Autodesk Inventor part; units mm, degrees
(part 5 of 6)
sketch "S12_252p5" plane through (0, 0, 0) normal (0, 0, 1) x (1, 0, 0)
  spline S0 degree 4 poles (166.9793, -57.9524) (166.9462, -57.9325) (166.7851, -57.8344) (166.5141, -57.6708) (166.0568, -57.3944) (165.5757, -57.1034) (164.9842, -56.7476) (164.2877, -56.3279) (163.4842, -55.8462) (162.5759, -55.3021) (161.5628, -54.6978) (160.4459, -54.033) (159.2262, -53.3098) (157.9042, -52.5289) (156.4819, -51.6916) (154.959, -50.7997) (153.338, -49.8542) (151.6196, -48.8571) (149.8054, -47.8089) (147.8966, -46.7125) (145.8951, -45.5691) (143.8025, -44.3805) (141.6201, -43.1481) (139.3507, -41.8743) (136.9951, -40.5607) (134.5563, -39.2099) (132.0355, -37.8225) (129.4358, -36.4019) (126.7586, -34.949) (124.007, -33.4672) (121.1827, -31.9571) (118.2887, -30.4221) (115.3274, -28.8634) (112.3016, -27.2839) (109.2136, -25.6852) (106.0671, -24.0697) (102.8636, -22.4398) (99.6073, -20.7974) (96.3005, -19.1452) (92.9462, -17.4849) (89.5478, -15.8193) (86.108, -14.1502) (82.6304, -12.4799) (79.1182, -10.811) (75.574, -9.1458) (72.0022, -7.4865) (68.4051, -5.8346) (64.7867, -4.1941) (61.15, -2.5653) (57.4989, -0.952) (53.8362, 0.6448) (50.1662, 2.222) (46.4912, 3.7772) (42.8159, 5.3099) (39.1427, 6.8159) (35.4729, 8.2959) (31.8154, 9.7442) (28.1539, 11.1682) (24.4959, 12.5514) (20.856, 13.8924) (17.2349, 15.189) (13.6386, 16.4388) (10.0712, 17.6417) (6.5362, 18.794) (3.0374, 19.8976) (-0.4212, 20.9484) (-3.8363, 21.9476) (-7.2038, 22.8929) (-10.5204, 23.7851) (-13.7822, 24.6219) (-16.9859, 25.4043) (-20.1277, 26.131) (-23.204, 26.8025) (-26.2119, 27.4178) (-29.1474, 27.978) (-32.0075, 28.4823) (-34.7892, 28.9318) (-37.4891, 29.3257) (-40.1042, 29.666) (-42.6316, 29.9518) (-45.0687, 30.184) (-47.4123, 30.3643) (-49.6602, 30.492) (-51.8096, 30.5686) (-53.8586, 30.5956) (-55.8044, 30.5726) (-57.6453, 30.5014) (-59.3792, 30.3829) (-61.0045, 30.2176) (-62.5192, 30.0064) (-63.9224, 29.7508) (-65.2124, 29.4515) (-66.3881, 29.1083) (-67.4495, 28.7237) (-68.3947, 28.2959) (-69.2243, 27.8264) (-69.9371, 27.3151) (-70.5323, 26.7606) (-71.007, 26.1624) (-71.3603, 25.5232) (-71.5883, 24.8429) (-71.6921, 24.1329) (-71.6666, 23.4034) (-71.5144, 22.6557) (-71.2376, 21.8925) (-70.8384, 21.1138) (-70.3185, 20.32) (-69.6791, 19.5098) (-68.9214, 18.6836) (-68.046, 17.8415) (-67.0539, 16.9836) (-65.9464, 16.1108) (-64.7243, 15.223) (-63.3893, 14.3214) (-61.9425, 13.406) (-60.3859, 12.4783) (-58.7208, 11.5376) (-56.9491, 10.5863) (-55.0727, 9.6235) (-53.0939, 8.6504) (-51.014, 7.6678) (-48.8358, 6.6768) (-46.5615, 5.676) (-44.1931, 4.6688) (-41.7338, 3.6529) (-39.1849, 2.6307) (-36.5503, 1.6015) (-33.832, 0.5658) (-31.0327, -0.4749) (-28.1557, -1.5226) (-25.2032, -2.5742) (-22.1791, -3.6324) (-19.0858, -4.6945) (-15.9263, -5.762) (-12.7047, -6.8345) (-9.4228, -7.9111) (-6.0855, -8.9929) (-2.695, -10.0789) (0.7449, -11.1692) (4.2307, -12.2643) (7.7587, -13.3643) (11.3259, -14.4678) (14.9302, -15.5774) (18.5666, -16.6895) (22.2391, -17.8119) (25.9566, -18.935) (29.6926, -20.0539) (33.4519, -21.1684) (37.2253, -22.2781) (41.0102, -23.3826) (44.8023, -24.4815) (48.5975, -25.5737) (52.392, -26.6597) (56.1823, -27.7377) (59.9639, -28.809) (63.7335, -29.871) (67.4868, -30.9251) (71.22, -31.9694) (74.9301, -33.0031) (78.6119, -34.0269) (82.2628, -35.0388) (85.8789, -36.0381) (89.4562, -37.0254) (92.9912, -37.9982) (96.4806, -38.9572) (99.9205, -39.9007) (103.3076, -40.8281) (106.6385, -41.7385) (109.9101, -42.6317) (113.1182, -43.5064) (116.2605, -44.3616) (119.3336, -45.1966) (122.3339, -46.0115) (125.2589, -46.8038) (128.1054, -47.5746) (130.8706, -48.3216) (133.5514, -49.0456) (136.1456, -49.7442) (138.65, -50.4184) (141.0622, -51.0663) (143.3799, -51.6882) (145.6004, -52.2825) (147.7216, -52.8503) (149.7413, -53.389) (151.6572, -53.9) (153.4675, -54.382) (155.1703, -54.8341) (156.7635, -55.2571) (158.2458, -55.6502) (159.6155, -56.0123) (160.8707, -56.3443) (162.0109, -56.6449) (163.0338, -56.915) (163.9393, -57.1532) (164.7255, -57.3602) (165.3927, -57.5359) (165.9368, -57.6783) (166.4534, -57.8147) (166.7596, -57.8945) (166.942, -57.9424) (166.9793, -57.9524) knots 0 0 0 0 0 0.003306 0.005253 0.00752 0.010062 0.01285 0.015861 0.019079 0.022488 0.026078 0.029837 0.033757 0.037828 0.042045 0.046398 0.050884 0.055494 0.060224 0.065069 0.070023 0.075082 0.080241 0.085495 0.090841 0.096274 0.101791 0.107386 0.113057 0.118799 0.124609 0.130484 0.136419 0.142412 0.148458 0.154554 0.160697 0.166884 0.17311 0.179374 0.185671 0.191998 0.198352 0.20473 0.211128 0.217543 0.223972 0.230412 0.23686 0.243312 0.249765 0.256217 0.262663 0.2691 0.275526 0.281941 0.288345 0.294734 0.301105 0.307451 0.313767 0.320049 0.326294 0.332498 0.338659 0.344773 0.350837 0.356848 0.362801 0.368695 0.374525 0.380288 0.38598 0.391599 0.39714 0.4026 0.407976 0.413263 0.418458 0.423557 0.428556 0.433452 0.438241 0.442917 0.447478 0.451919 0.456236 0.460425 0.464482 0.468403 0.472185 0.475825 0.479322 0.482675 0.485889 0.48897 0.49193 0.494788 0.497572 0.50031 0.503032 0.505769 0.508552 0.511409 0.514365 0.517441 0.520647 0.523991 0.527474 0.531098 0.534861 0.538758 0.542789 0.546947 0.551231 0.555634 0.560154 0.564786 0.569527 0.574371 0.579315 0.584356 0.58949 0.594712 0.60002 0.605409 0.610877 0.61642 0.622034 0.627716 0.633463 0.639271 0.645138 0.651061 0.657035 0.663059 0.669128 0.675241 0.681393 0.687582 0.693804 0.700057 0.706341 0.712655 0.718998 0.725365 0.731751 0.738149 0.744556 0.750969 0.757385 0.7638 0.770211 0.776616 0.783011 0.789393 0.795759 0.802106 0.808429 0.814727 0.820996 0.827232 0.833433 0.839595 0.845714 0.851788 0.857813 0.863785 0.869702 0.875558 0.881352 0.887078 0.892735 0.898316 0.90382 0.909242 0.914577 0.919822 0.924972 0.930023 0.93497 0.939808 0.944533 0.949139 0.95362 0.95797 0.962183 0.966252 0.970169 0.973927 0.977515 0.980924 0.984141 0.987151 0.989939 0.99248 0.994747 0.996694 1 1 1 1 1
  circle A0 centre (0, 0) radius 5.15
  line L0 (-56.62, 15.9) -> (-46.42, 15.9)
  line L1 (-46.42, 15.9) -> (-46.42, 20.1)
  line L2 (-46.42, 20.1) -> (-56.62, 20.1)
  line L3 (-56.62, 20.1) -> (-56.62, 15.9)
  line L4 (-56.62, 15.9) -> (-46.42, 20.1) construction
  line L5 (-46.42, 15.9) -> (-56.62, 20.1) construction
  line L6 (-30.35, 13.1) -> (-20.15, 13.1)
  line L7 (-20.15, 13.1) -> (-20.15, 8.9)
  line L8 (-20.15, 8.9) -> (-30.35, 8.9)
  line L9 (-30.35, 8.9) -> (-30.35, 13.1)
  line L10 (-30.35, 13.1) -> (-20.15, 8.9) construction
  line L11 (-20.15, 13.1) -> (-30.35, 8.9) construction
  line L12 (64.9, -14.9) -> (75.1, -14.9)
  line L13 (75.1, -14.9) -> (75.1, -19.1)
  line L14 (75.1, -19.1) -> (64.9, -19.1)
  line L15 (64.9, -19.1) -> (64.9, -14.9)
  line L16 (64.9, -14.9) -> (75.1, -19.1) construction
  line L17 (75.1, -14.9) -> (64.9, -19.1) construction
  line L18 (29.9, -6.2) -> (40.1, -6.2)
  line L19 (40.1, -6.2) -> (40.1, -10.4)
  line L20 (40.1, -10.4) -> (29.9, -10.4)
  line L21 (29.9, -10.4) -> (29.9, -6.2)
  line L22 (29.9, -6.2) -> (40.1, -10.4) construction
  line L23 (40.1, -6.2) -> (29.9, -10.4) construction
  point P0 (166.7636, -57.8216)
  point P1 (166.4938, -57.6585)
  point P2 (166.1167, -57.4306)
  point P3 (165.6324, -57.138)
  point P4 (165.041, -56.7817)
  point P5 (164.3433, -56.3618)
  point P6 (163.5394, -55.8794)
  point P7 (162.6303, -55.3351)
  point P8 (161.6167, -54.7302)
  point P9 (160.4991, -54.0652)
  point P10 (159.2787, -53.3415)
  point P11 (157.9561, -52.5601)
  point P12 (156.5328, -51.7224)
  point P13 (155.0093, -50.8299)
  point P14 (153.3873, -49.884)
  point P15 (151.6681, -48.8861)
  point P16 (149.8529, -47.8376)
  point P17 (147.9432, -46.7405)
  point P18 (145.9406, -45.5964)
  point P19 (143.8469, -44.4071)
  point P20 (141.6635, -43.1741)
  point P21 (139.3928, -41.8996)
  point P22 (137.0361, -40.5854)
  point P23 (134.5959, -39.2336)
  point P24 (132.074, -37.8457)
  point P25 (129.4729, -36.4241)
  point P26 (126.7943, -34.9707)
  point P27 (124.0413, -33.4878)
  point P28 (121.2155, -31.9771)
  point P29 (118.32, -30.4411)
  point P30 (115.3573, -28.8818)
  point P31 (112.3299, -27.3014)
  point P32 (109.2405, -25.7018)
  point P33 (106.0922, -24.0856)
  point P34 (102.8872, -22.4547)
  point P35 (99.629, -20.8116)
  point P36 (96.3206, -19.1584)
  point P37 (92.9647, -17.4974)
  point P38 (89.5644, -15.8309)
  point P39 (86.1228, -14.1609)
  point P40 (82.6434, -12.4899)
  point P41 (79.1293, -10.8202)
  point P42 (75.5835, -9.1542)
  point P43 (72.0097, -7.494)
  point P44 (68.4108, -5.8416)
  point P45 (64.7904, -4.2)
  point P46 (61.1519, -2.5707)
  point P47 (57.4988, -0.9565)
  point P48 (53.8343, 0.6409)
  point P49 (50.1622, 2.2187)
  point P50 (46.4854, 3.7749)
  point P51 (42.8081, 5.3077)
  point P52 (39.1333, 6.8146)
  point P53 (35.4648, 8.2936)
  point P54 (31.8059, 9.7425)
  point P55 (28.1423, 11.1645)
  point P56 (24.4805, 12.5497)
  point P57 (20.8364, 13.8917)
  point P58 (17.2133, 15.1887)
  point P59 (13.6151, 16.4391)
  point P60 (10.0459, 17.6418)
  point P61 (6.5091, 18.795)
  point P62 (3.0085, 19.8982)
  point P63 (-0.4519, 20.9495)
  point P64 (-3.8686, 21.9485)
  point P65 (-7.2379, 22.8941)
  point P66 (-10.5561, 23.786)
  point P67 (-13.8196, 24.623)
  point P68 (-17.0248, 25.4051)
  point P69 (-20.1681, 26.1317)
  point P70 (-23.246, 26.8027)
  point P71 (-26.2553, 27.4179)
  point P72 (-29.1922, 27.9775)
  point P73 (-32.0535, 28.4814)
  point P74 (-34.8365, 28.9301)
  point P75 (-37.5376, 29.3237)
  point P76 (-40.1538, 29.6629)
  point P77 (-42.6822, 29.9479)
  point P78 (-45.1201, 30.1792)
  point P79 (-47.4646, 30.3581)
  point P80 (-49.7131, 30.4847)
  point P81 (-51.8631, 30.5601)
  point P82 (-53.9124, 30.5852)
  point P83 (-55.8584, 30.5606)
  point P84 (-57.6991, 30.4874)
  point P85 (-59.4326, 30.3666)
  point P86 (-61.0571, 30.1989)
  point P87 (-62.5705, 29.9851)
  point P88 (-63.9718, 29.7266)
  point P89 (-65.259, 29.4239)
  point P90 (-66.4311, 29.0778)
  point P91 (-67.4872, 28.6895)
  point P92 (-68.4258, 28.2591)
  point P93 (-69.2466, 27.7879)
  point P94 (-69.9487, 27.2765)
  point P95 (-70.5316, 26.7251)
  point P96 (-70.9949, 26.1343)
  point P97 (-71.3387, 25.5047)
  point P98 (-71.5626, 24.8367)
  point P99 (-71.6647, 24.1396)
  point P100 (-71.643, 23.4227)
  point P101 (-71.4981, 22.6866)
  point P102 (-71.2305, 21.9314)
  point P103 (-70.8405, 21.1575)
  point P104 (-70.329, 20.3658)
  point P105 (-69.6967, 19.5562)
  point P106 (-68.9447, 18.7294)
  point P107 (-68.074, 17.886)
  point P108 (-67.0856, 17.0266)
  point P109 (-65.9809, 16.1519)
  point P110 (-64.7611, 15.2624)
  point P111 (-63.4277, 14.3589)
  point P112 (-61.9822, 13.4419)
  point P113 (-60.4264, 12.5123)
  point P114 (-58.7619, 11.5703)
  point P115 (-56.9906, 10.6171)
  point P116 (-55.1143, 9.653)
  point P117 (-53.1352, 8.6785)
  point P118 (-51.0552, 7.6947)
  point P119 (-48.8766, 6.7021)
  point P120 (-46.6017, 5.7006)
  point P121 (-44.2329, 4.6916)
  point P122 (-41.7726, 3.675)
  point P123 (-39.2231, 2.6514)
  point P124 (-36.5875, 1.6212)
  point P125 (-33.8682, 0.5847)
  point P126 (-31.068, -0.4574)
  point P127 (-28.1897, -1.5055)
  point P128 (-25.2362, -2.5587)
  point P129 (-22.2108, -3.6172)
  point P130 (-19.1162, -4.6805)
  point P131 (-15.9555, -5.7489)
  point P132 (-12.7324, -6.8221)
  point P133 (-9.4493, -7.8998)
  point P134 (-6.1103, -8.9822)
  point P135 (-2.7184, -10.0691)
  point P136 (0.723, -11.1603)
  point P137 (4.2104, -12.2562)
  point P138 (7.74, -13.3567)
  point P139 (11.3086, -14.4613)
  point P140 (14.9124, -15.5704)
  point P141 (18.5481, -16.6836)
  point P142 (22.2237, -17.8045)
  point P143 (25.9431, -18.9289)
  point P144 (29.6848, -20.0492)
  point P145 (33.4457, -21.1647)
  point P146 (37.2213, -22.2752)
  point P147 (41.008, -23.3804)
  point P148 (44.802, -24.4799)
  point P149 (48.5991, -25.5729)
  point P150 (52.3956, -26.6593)
  point P151 (56.1876, -27.7383)
  point P152 (59.9713, -28.8099)
  point P153 (63.7427, -29.8729)
  point P154 (67.4979, -30.9274)
  point P155 (71.2331, -31.9722)
  point P156 (74.9449, -33.0068)
  point P157 (78.6288, -34.0309)
  point P158 (82.2815, -35.0434)
  point P159 (85.8994, -36.0435)
  point P160 (89.4786, -37.031)
  point P161 (93.0154, -38.0046)
  point P162 (96.5066, -38.9639)
  point P163 (99.9484, -39.908)
  point P164 (103.3372, -40.8358)
  point P165 (106.6699, -41.7469)
  point P166 (109.9431, -42.6405)
  point P167 (113.153, -43.5155)
  point P168 (116.2969, -44.3712)
  point P169 (119.3716, -45.2069)
  point P170 (122.3736, -46.0218)
  point P171 (125.3, -46.8148)
  point P172 (128.1481, -47.5857)
  point P173 (130.9147, -48.3334)
  point P174 (133.597, -49.0575)
  point P175 (136.1925, -49.7568)
  point P176 (138.6983, -50.4311)
  point P177 (141.1118, -51.0795)
  point P178 (143.4308, -51.7015)
  point P179 (145.6525, -52.2964)
  point P180 (147.7749, -52.8641)
  point P181 (149.7956, -53.4035)
  point P182 (151.7126, -53.9146)
  point P183 (153.5239, -54.3967)
  point P184 (155.2276, -54.8493)
  point P185 (156.8218, -55.2724)
  point P186 (158.305, -55.6656)
  point P187 (159.6754, -56.0282)
  point P188 (160.9315, -56.3602)
  point P189 (162.0723, -56.6612)
  point P190 (163.0961, -56.9312)
  point P191 (164.0022, -57.1698)
  point P192 (164.7895, -57.377)
  point P193 (165.4569, -57.5526)
  point P194 (166.0044, -57.6963)
  point P195 (166.4306, -57.8084)
  point P196 (166.7353, -57.8883)
  point P197 (166.9183, -57.9363)
  point P198 (-51.52, 18)
  point P199 (-25.25, 11)
  dimension "d23" = 10.3
  dimension "d24" = 75.75
  dimension "d106" = 10.2
  dimension "d107" = 4.2
  dimension "d109" = 10.2
  dimension "d110" = 4.2
  dimension "d169" = 51.52
  dimension "d170" = 18
  dimension "d172" = 25.25
  dimension "d173" = 11
  dimension "d275" = 10.2
  dimension "d276" = 4.2
  dimension "d277" = 70
  dimension "d278" = 17
  dimension "d279" = 10.2
  dimension "d280" = 4.2
  dimension "d281" = 35
  dimension "d282" = 8.3
  constraints: 48 end point, 8 midpoint, 8 parallel, 4 horizontal, 4 perpendicular, 1 centre point, 201 other
  measures "d23" diameter of A0
  measures "d24" distance of A0.centre point (-71.563, 24.837)
  measures "d106" distance of L2.end L1.end
  measures "d107" distance of L1.end L0.end
  measures "d109" distance of L7.end L8.end
  measures "d110" distance of L6.end L7.end
  measures "d169" horizontal distance of point (0, 0) point (-51.52, 18)
  measures "d170" vertical distance of point (0, 0) point (-51.52, 18)
  measures "d172" horizontal distance of point (0, 0) point (-25.25, 11)
  measures "d173" vertical distance of point (0, 0) point (-25.25, 11)
  measures "d275" distance of L13.end L14.end
  measures "d276" distance of L12.end L13.end
  measures "d277" horizontal distance of point (0, 0) point (70, -17)
  measures "d278" vertical distance of point (0, 0) point (70, -17)
  measures "d279" distance of L19.end L20.end
  measures "d280" distance of L18.end L19.end
  measures "d281" horizontal distance of point (0, 0) point (35, -8.3)
  measures "d282" vertical distance of point (0, 0) point (35, -8.3)
sketch "S13_240p0" plane through (0, 0, 0) normal (0, 0, 1) x (1, 0, 0)
  spline S0 degree 4 poles (158.1572, -56.6596) (158.1259, -56.6404) (157.9737, -56.5456) (157.7176, -56.3876) (157.2856, -56.1206) (156.8312, -55.8394) (156.2723, -55.4957) (155.6143, -55.0902) (154.8551, -54.6248) (153.9971, -54.099) (153.0398, -53.5152) (151.9845, -52.8727) (150.8321, -52.1738) (149.583, -51.4191) (148.2391, -50.6098) (146.8001, -49.7478) (145.2684, -48.8338) (143.6445, -47.8698) (141.9302, -46.8564) (140.1263, -45.7963) (138.2348, -44.6906) (136.2571, -43.5411) (134.1946, -42.3492) (132.0497, -41.117) (129.8232, -39.8462) (127.518, -38.5393) (125.1353, -37.1968) (122.6778, -35.8221) (120.147, -34.4158) (117.5457, -32.9814) (114.8756, -31.5194) (112.1396, -30.0331) (109.3397, -28.5237) (106.4788, -26.9939) (103.559, -25.4451) (100.5837, -23.8799) (97.5544, -22.3005) (94.4749, -20.7087) (91.3476, -19.1071) (88.1752, -17.4974) (84.9609, -15.8821) (81.7073, -14.2632) (78.4179, -12.6429) (75.0955, -11.0234) (71.7427, -9.4073) (68.3636, -7.7964) (64.9603, -6.1923) (61.5367, -4.5989) (58.0957, -3.0164) (54.6407, -1.4485) (51.1746, 0.1038) (47.7013, 1.6376) (44.2232, 3.1504) (40.7445, 4.6419) (37.2676, 6.108) (33.7936, 7.5494) (30.331, 8.9605) (26.8644, 10.3486) (23.4007, 11.6978) (19.9539, 13.0068) (16.5245, 14.2734) (13.1183, 15.4953) (9.739, 16.6722) (6.3901, 17.8009) (3.0751, 18.883) (-0.2022, 19.9143) (-3.4386, 20.8963) (-6.6304, 21.8267) (-9.7742, 22.706) (-12.8665, 23.5322) (-15.904, 24.3061) (-18.8832, 25.0265) (-21.8007, 25.6938) (-24.6538, 26.3071) (-27.4386, 26.8673) (-30.1521, 27.3736) (-32.7918, 27.8271) (-35.3541, 28.2271) (-37.8365, 28.5752) (-40.2359, 28.8708) (-42.5501, 29.1144) (-44.7758, 29.308) (-46.9111, 29.4507) (-48.9533, 29.5438) (-50.9005, 29.5888) (-52.7501, 29.5853) (-54.5004, 29.5351) (-56.1495, 29.4388) (-57.6959, 29.2971) (-59.1375, 29.1107) (-60.4736, 28.8811) (-61.7025, 28.6087) (-62.8232, 28.2936) (-63.8357, 27.9382) (-64.7381, 27.5405) (-65.531, 27.1021) (-66.2133, 26.6229) (-66.7842, 26.1015) (-67.2411, 25.5374) (-67.5829, 24.9332) (-67.806, 24.2888) (-67.9114, 23.615) (-67.8941, 22.9213) (-67.7565, 22.2093) (-67.5007, 21.4813) (-67.1286, 20.7374) (-66.6419, 19.978) (-66.0418, 19.2019) (-65.3295, 18.4095) (-64.5055, 17.6008) (-63.5707, 16.7761) (-62.5263, 15.936) (-61.3731, 15.0807) (-60.1128, 14.2112) (-58.7464, 13.3274) (-57.2757, 12.431) (-55.702, 11.5211) (-54.0271, 10.6002) (-52.2528, 9.6674) (-50.3812, 8.7238) (-48.4136, 7.7703) (-46.3527, 6.8078) (-44.2006, 5.8351) (-41.9591, 4.8553) (-39.6312, 3.8665) (-37.2184, 2.8708) (-34.724, 1.8678) (-32.1502, 0.8576) (-29.4995, -0.158) (-26.7749, -1.181) (-23.9787, -2.2084) (-21.1145, -3.2426) (-18.1844, -4.2814) (-15.1916, -5.3259) (-12.1398, -6.3757) (-9.0307, -7.43) (-5.869, -8.4897) (-2.6568, -9.554) (0.6023, -10.6228) (3.905, -11.6966) (7.2479, -12.7754) (10.6279, -13.858) (14.0431, -14.9467) (17.4888, -16.038) (20.9687, -17.1395) (24.4913, -18.2422) (28.0316, -19.3409) (31.5941, -20.4358) (35.17, -21.5262) (38.757, -22.6118) (42.3508, -23.692) (45.9476, -24.766) (49.5438, -25.8341) (53.1361, -26.8945) (56.7202, -27.9485) (60.293, -28.9935) (63.8502, -30.0309) (67.3886, -31.0587) (70.9051, -32.0763) (74.3948, -33.0841) (77.8552, -34.0804) (81.2826, -35.0644) (84.6734, -36.0366) (88.024, -36.9946) (91.3314, -37.9391) (94.592, -38.8684) (97.8025, -39.7818) (100.9597, -40.6786) (104.0607, -41.5585) (107.1016, -42.4202) (110.0801, -43.2627) (112.993, -44.0854) (115.8369, -44.8883) (118.6095, -45.6689) (121.3077, -46.4285) (123.9288, -47.1646) (126.4699, -47.8782) (128.9289, -48.5666) (131.3029, -49.2311) (133.5894, -49.8697) (135.7864, -50.4827) (137.8913, -51.0686) (139.902, -51.6283) (141.8165, -52.1594) (143.6326, -52.6632) (145.3486, -53.1384) (146.9628, -53.5842) (148.473, -54.0013) (149.8782, -54.3889) (151.1766, -54.746) (152.3665, -55.0735) (153.4473, -55.37) (154.417, -55.6364) (155.2754, -55.8713) (156.0207, -56.0755) (156.6531, -56.2488) (157.1689, -56.3893) (157.6586, -56.5238) (157.9489, -56.6025) (158.1218, -56.6498) (158.1572, -56.6596) knots 0 0 0 0 0 0.003306 0.005253 0.00752 0.010062 0.01285 0.015861 0.019079 0.022488 0.026078 0.029837 0.033757 0.037828 0.042045 0.046398 0.050884 0.055494 0.060224 0.065069 0.070023 0.075082 0.080241 0.085495 0.090841 0.096274 0.101791 0.107386 0.113057 0.118799 0.124609 0.130484 0.136419 0.142412 0.148458 0.154554 0.160697 0.166884 0.17311 0.179374 0.185671 0.191998 0.198352 0.20473 0.211128 0.217543 0.223972 0.230412 0.23686 0.243312 0.249765 0.256217 0.262663 0.2691 0.275526 0.281941 0.288345 0.294734 0.301105 0.307451 0.313767 0.320049 0.326294 0.332498 0.338659 0.344773 0.350837 0.356848 0.362801 0.368695 0.374525 0.380288 0.38598 0.391599 0.39714 0.4026 0.407976 0.413263 0.418458 0.423557 0.428556 0.433452 0.438241 0.442917 0.447478 0.451919 0.456236 0.460425 0.464482 0.468403 0.472185 0.475825 0.479322 0.482675 0.485889 0.48897 0.49193 0.494788 0.497572 0.50031 0.503032 0.505769 0.508552 0.511409 0.514365 0.517441 0.520647 0.523991 0.527474 0.531098 0.534861 0.538758 0.542789 0.546947 0.551231 0.555634 0.560154 0.564786 0.569527 0.574371 0.579315 0.584356 0.58949 0.594712 0.60002 0.605409 0.610877 0.61642 0.622034 0.627716 0.633463 0.639271 0.645138 0.651061 0.657035 0.663059 0.669128 0.675241 0.681393 0.687582 0.693804 0.700057 0.706341 0.712655 0.718998 0.725365 0.731751 0.738149 0.744556 0.750969 0.757385 0.7638 0.770211 0.776616 0.783011 0.789393 0.795759 0.802106 0.808429 0.814727 0.820996 0.827232 0.833433 0.839595 0.845714 0.851788 0.857813 0.863785 0.869702 0.875558 0.881352 0.887078 0.892735 0.898316 0.90382 0.909242 0.914577 0.919822 0.924972 0.930023 0.93497 0.939808 0.944533 0.949139 0.95362 0.95797 0.962183 0.966252 0.970169 0.973927 0.977515 0.980924 0.984141 0.987151 0.989939 0.99248 0.994747 0.996694 1 1 1 1 1
  circle A0 centre (0, 0) radius 5.15
  line L0 (-47.1, 22.1) -> (-36.9, 22.1)
  line L1 (-36.9, 22.1) -> (-36.9, 17.9)
  line L2 (-36.9, 17.9) -> (-47.1, 17.9)
  line L3 (-47.1, 17.9) -> (-47.1, 22.1)
  line L4 (-47.1, 22.1) -> (-36.9, 17.9) construction
  line L5 (-36.9, 22.1) -> (-47.1, 17.9) construction
  line L6 (-30.35, 8.9) -> (-20.15, 8.9)
  line L7 (-20.15, 8.9) -> (-20.15, 13.1)
  line L8 (-20.15, 13.1) -> (-30.35, 13.1)
  line L9 (-30.35, 13.1) -> (-30.35, 8.9)
  line L10 (-30.35, 8.9) -> (-20.15, 13.1) construction
  line L11 (-20.15, 8.9) -> (-30.35, 13.1) construction
  line L12 (29.9, -6.2) -> (40.1, -6.2)
  line L13 (40.1, -6.2) -> (40.1, -10.4)
  line L14 (40.1, -10.4) -> (29.9, -10.4)
  line L15 (29.9, -10.4) -> (29.9, -6.2)
  line L16 (29.9, -6.2) -> (40.1, -10.4) construction
  line L17 (40.1, -6.2) -> (29.9, -10.4) construction
  line L18 (54.9, -17.9) -> (65.1, -17.9)
  line L19 (65.1, -17.9) -> (65.1, -22.1)
  line L20 (65.1, -22.1) -> (54.9, -22.1)
  line L21 (54.9, -22.1) -> (54.9, -17.9)
  line L22 (54.9, -17.9) -> (65.1, -22.1) construction
  line L23 (65.1, -17.9) -> (54.9, -22.1) construction
  point P0 (157.9533, -56.5333)
  point P1 (157.6985, -56.3757)
  point P2 (157.3422, -56.1555)
  point P3 (156.8847, -55.8728)
  point P4 (156.326, -55.5287)
  point P5 (155.6668, -55.123)
  point P6 (154.9073, -54.6569)
  point P7 (154.0485, -54.131)
  point P8 (153.0908, -53.5464)
  point P9 (152.0348, -52.9038)
  point P10 (150.8817, -52.2044)
  point P11 (149.6321, -51.4492)
  point P12 (148.2872, -50.6396)
  point P13 (146.8477, -49.7769)
  point P14 (145.315, -48.8625)
  point P15 (143.6904, -47.8979)
  point P16 (141.9751, -46.8841)
  point P17 (140.1703, -45.8233)
  point P18 (138.2778, -44.717)
  point P19 (136.2991, -43.5668)
  point P20 (134.2356, -42.3743)
  point P21 (132.0894, -41.1415)
  point P22 (129.8619, -39.8701)
  point P23 (127.5555, -38.5622)
  point P24 (125.1716, -37.2192)
  point P25 (122.7128, -35.8435)
  point P26 (120.1807, -34.4367)
  point P27 (117.5781, -33.0014)
  point P28 (114.9067, -31.5388)
  point P29 (112.1692, -30.0515)
  point P30 (109.368, -28.5414)
  point P31 (106.5056, -27.0107)
  point P32 (103.5844, -25.4612)
  point P33 (100.6074, -23.8953)
  point P34 (97.5766, -22.3149)
  point P35 (94.4954, -20.7224)
  point P36 (91.3666, -19.1199)
  point P37 (88.1926, -17.5094)
  point P38 (84.9766, -15.8933)
  point P39 (81.7214, -14.2736)
  point P40 (78.4302, -12.6525)
  point P41 (75.106, -11.0323)
  point P42 (71.7516, -9.4153)
  point P43 (68.3706, -7.8035)
  point P44 (64.9656, -6.199)
  point P45 (61.5402, -4.6045)
  point P46 (58.0974, -3.0216)
  point P47 (54.6406, -1.4528)
  point P48 (51.1728, 0.1001)
  point P49 (47.6975, 1.6344)
  point P50 (44.2177, 3.1482)
  point P51 (40.7371, 4.6399)
  point P52 (37.2586, 6.1069)
  point P53 (33.7859, 7.5472)
  point P54 (30.322, 8.959)
  point P55 (26.8533, 10.3452)
  point P56 (23.3862, 11.6964)
  point P57 (19.9353, 13.0063)
  point P58 (16.504, 14.2733)
  point P59 (13.0959, 15.4958)
  point P60 (9.7149, 16.6726)
  point P61 (6.3643, 17.8021)
  point P62 (3.0476, 18.8837)
  point P63 (-0.2314, 19.9157)
  point P64 (-3.4694, 20.8975)
  point P65 (-6.6628, 21.8281)
  point P66 (-9.8081, 22.7071)
  point P67 (-12.902, 23.5335)
  point P68 (-15.941, 24.3072)
  point P69 (-18.9217, 25.0275)
  point P70 (-21.8406, 25.6944)
  point P71 (-24.695, 26.3075)
  point P72 (-27.4811, 26.8672)
  point P73 (-30.1959, 27.3732)
  point P74 (-32.8367, 27.826)
  point P75 (-35.4002, 28.2256)
  point P76 (-37.8836, 28.5727)
  point P77 (-40.284, 28.8675)
  point P78 (-42.599, 29.1104)
  point P79 (-44.8256, 29.3026)
  point P80 (-46.9614, 29.4442)
  point P81 (-49.0042, 29.5362)
  point P82 (-50.9517, 29.5794)
  point P83 (-52.8015, 29.5745)
  point P84 (-54.5517, 29.5223)
  point P85 (-56.2005, 29.4239)
  point P86 (-57.746, 29.2798)
  point P87 (-59.1865, 29.091)
  point P88 (-60.5208, 28.8585)
  point P89 (-61.7471, 28.5829)
  point P90 (-62.8644, 28.2651)
  point P91 (-63.8718, 27.906)
  point P92 (-64.768, 27.5059)
  point P93 (-65.5525, 27.0657)
  point P94 (-66.2247, 26.5863)
  point P95 (-66.784, 26.0678)
  point P96 (-67.2298, 25.5106)
  point P97 (-67.5626, 24.9155)
  point P98 (-67.7816, 24.2827)
  point P99 (-67.8853, 23.6211)
  point P100 (-67.8715, 22.9395)
  point P101 (-67.7408, 22.2385)
  point P102 (-67.4935, 21.5182)
  point P103 (-67.1302, 20.779)
  point P104 (-66.6515, 20.0216)
  point P105 (-66.0582, 19.2462)
  point P106 (-65.3513, 18.4533)
  point P107 (-64.5317, 17.6434)
  point P108 (-63.6004, 16.8172)
  point P109 (-62.5587, 15.9755)
  point P110 (-61.4077, 15.1185)
  point P111 (-60.149, 14.2472)
  point P112 (-58.7838, 13.3619)
  point P113 (-57.3139, 12.4636)
  point P114 (-55.7407, 11.5526)
  point P115 (-54.0662, 10.6299)
  point P116 (-52.292, 9.6958)
  point P117 (-50.4202, 8.7509)
  point P118 (-48.4525, 7.7962)
  point P119 (-46.3913, 6.8321)
  point P120 (-44.2386, 5.8587)
  point P121 (-41.9967, 4.8774)
  point P122 (-39.668, 3.8879)
  point P123 (-37.2545, 2.8909)
  point P124 (-34.7592, 1.8868)
  point P125 (-32.1844, 0.876)
  point P126 (-29.5329, -0.141)
  point P127 (-26.8071, -1.1644)
  point P128 (-24.0099, -2.1932)
  point P129 (-21.1444, -3.228)
  point P130 (-18.2133, -4.2679)
  point P131 (-15.2193, -5.3132)
  point P132 (-12.166, -6.3637)
  point P133 (-9.0557, -7.419)
  point P134 (-5.8925, -8.4793)
  point P135 (-2.6789, -9.5444)
  point P136 (0.5816, -10.6141)
  point P137 (3.8859, -11.6887)
  point P138 (7.2302, -12.768)
  point P139 (10.6115, -13.8516)
  point P140 (14.0263, -14.9399)
  point P141 (17.4712, -16.0323)
  point P142 (20.9542, -17.1324)
  point P143 (24.4786, -18.2362)
  point P144 (28.0243, -19.3364)
  point P145 (31.5883, -20.4322)
  point P146 (35.1663, -21.5233)
  point P147 (38.7549, -22.6096)
  point P148 (42.3505, -23.6905)
  point P149 (45.9491, -24.7653)
  point P150 (49.5472, -25.8337)
  point P151 (53.1411, -26.8951)
  point P152 (56.7272, -27.9494)
  point P153 (60.3017, -28.9954)
  point P154 (63.8608, -30.0331)
  point P155 (67.401, -31.0615)
  point P156 (70.9191, -32.0799)
  point P157 (74.4108, -33.0881)
  point P158 (77.8729, -34.0849)
  point P159 (81.3021, -35.0697)
  point P160 (84.6946, -36.0421)
  point P161 (88.047, -37.0009)
  point P162 (91.3561, -37.9457)
  point P163 (94.6184, -38.8756)
  point P164 (97.8305, -39.7895)
  point P165 (100.9894, -40.6869)
  point P166 (104.092, -41.5671)
  point P167 (107.1345, -42.4292)
  point P168 (110.1146, -43.2722)
  point P169 (113.029, -44.0955)
  point P170 (115.8745, -44.8985)
  point P171 (118.6485, -45.6799)
  point P172 (121.3481, -46.4395)
  point P173 (123.9706, -47.1763)
  point P174 (126.5131, -47.8899)
  point P175 (128.9734, -48.579)
  point P176 (131.3487, -49.2436)
  point P177 (133.6364, -49.8827)
  point P178 (135.8346, -50.4958)
  point P179 (137.9406, -51.0823)
  point P180 (139.9524, -51.6419)
  point P181 (141.868, -52.1737)
  point P182 (143.6851, -52.6776)
  point P183 (145.4021, -53.153)
  point P184 (147.0171, -53.5992)
  point P185 (148.5283, -54.0164)
  point P186 (149.9343, -54.4042)
  point P187 (151.2334, -54.7617)
  point P188 (152.4241, -55.0891)
  point P189 (153.5055, -55.386)
  point P190 (154.476, -55.6524)
  point P191 (155.335, -55.8877)
  point P192 (156.0813, -56.0921)
  point P193 (156.714, -56.2652)
  point P194 (157.233, -56.407)
  point P195 (157.637, -56.5176)
  point P196 (157.9259, -56.5964)
  point P197 (158.0994, -56.6437)
  point P198 (-42, 20)
  point P199 (-25.25, 11)
  dimension "d25" = 10.3
  dimension "d26" = 72
  dimension "d112" = 10.2
  dimension "d113" = 4.2
  dimension "d114" = 10.2
  dimension "d115" = 4.2
  dimension "d174" = 25.25
  dimension "d175" = 11
  dimension "d176" = 42
  dimension "d177" = 20
  dimension "d283" = 10.2
  dimension "d284" = 4.2
  dimension "d285" = 35
  dimension "d286" = 8.3
  dimension "d287" = 10.2
  dimension "d288" = 4.2
  dimension "d289" = 60
  dimension "d290" = 20
  constraints: 48 end point, 8 midpoint, 8 parallel, 4 horizontal, 4 perpendicular, 1 centre point, 201 other
  measures "d25" diameter of A0
  measures "d26" distance of A0.centre point (-67.782, 24.283)
  measures "d112" distance of L1.end L2.end
  measures "d113" distance of L0.end L1.end
  measures "d114" distance of L8.end L7.end
  measures "d115" distance of L7.end L6.end
  measures "d174" horizontal distance of point (0, 0) point (-25.25, 11)
  measures "d175" vertical distance of point (0, 0) point (-25.25, 11)
  measures "d176" horizontal distance of point (0, 0) point (-42, 20)
  measures "d177" vertical distance of point (0, 0) point (-42, 20)
  measures "d283" distance of L13.end L14.end
  measures "d284" distance of L12.end L13.end
  measures "d285" horizontal distance of point (0, 0) point (35, -8.3)
  measures "d286" vertical distance of point (0, 0) point (35, -8.3)
  measures "d287" distance of L19.end L20.end
  measures "d288" distance of L18.end L19.end
  measures "d289" horizontal distance of point (60, -20) point (0, 0)
  measures "d290" vertical distance of point (0, 0) point (60, -20)
sketch "S14_219p8" plane through (0, 0, 0) normal (0, 0, 1) x (1, 0, 0)
  spline S0 degree 4 poles (141.7858, -59.7469) (141.7582, -59.7278) (141.6237, -59.6335) (141.3975, -59.4761) (141.0158, -59.2103) (140.6143, -58.9304) (140.1205, -58.588) (139.5392, -58.1842) (138.8683, -57.7205) (138.11, -57.1966) (137.2639, -56.6147) (136.3311, -55.9743) (135.3124, -55.2774) (134.208, -54.5246) (133.0196, -53.7171) (131.747, -52.8566) (130.3921, -51.9439) (128.9555, -50.981) (127.4387, -49.9683) (125.8423, -48.9083) (124.1681, -47.8023) (122.4172, -46.652) (120.5909, -45.4585) (118.6912, -44.2242) (116.719, -42.9504) (114.6765, -41.6396) (112.565, -40.2924) (110.3867, -38.912) (108.1429, -37.499) (105.8361, -36.0569) (103.4678, -34.586) (101.0403, -33.0896) (98.5557, -31.5688) (96.0163, -30.0263) (93.4239, -28.4636) (90.7816, -26.8831) (88.0907, -25.2868) (85.3545, -23.6766) (82.575, -22.0552) (79.7548, -20.424) (76.8965, -18.7857) (74.0024, -17.142) (71.0756, -15.4953) (68.1187, -13.8477) (65.1338, -12.2016) (62.1245, -10.559) (59.0929, -8.9214) (56.0421, -7.2925) (52.9747, -5.6728) (49.894, -4.0657) (46.8023, -2.4723) (43.703, -0.8955) (40.5983, 0.6624) (37.492, 2.2009) (34.3861, 3.716) (31.2815, 5.2083) (28.1859, 6.6725) (25.0856, 8.1157) (21.9858, 9.5233) (18.8995, 10.8932) (15.827, 12.2235) (12.7734, 13.5117) (9.7423, 14.7575) (6.7365, 15.9577) (3.7593, 17.1134) (0.8141, 18.2209) (-2.0962, 19.2813) (-4.9683, 20.2922) (-7.799, 21.254) (-10.5853, 22.1647) (-13.3242, 23.0248) (-16.0125, 23.833) (-18.6469, 24.5896) (-21.2252, 25.2935) (-23.7436, 25.9455) (-26.1996, 26.5446) (-28.5907, 27.0918) (-30.9138, 27.586) (-33.1664, 28.0289) (-35.3457, 28.4196) (-37.4497, 28.7585) (-39.4754, 29.0471) (-41.4208, 29.2847) (-43.2837, 29.4723) (-45.062, 29.6112) (-46.7536, 29.7008) (-48.3567, 29.7426) (-49.8696, 29.7373) (-51.2908, 29.6853) (-52.6184, 29.5872) (-53.8518, 29.4442) (-54.9892, 29.2568) (-56.0299, 29.0249) (-56.9735, 28.7507) (-57.8187, 28.4322) (-58.5657, 28.0712) (-59.2137, 27.6671) (-59.762, 27.219) (-60.2081, 26.7261) (-60.551, 26.1907) (-60.7873, 25.6126) (-60.9175, 25.0018) (-60.9364, 24.3666) (-60.8464, 23.7085) (-60.6489, 23.0299) (-60.346, 22.331) (-59.939, 21.6122) (-59.4292, 20.8724) (-58.8176, 20.1121) (-58.1046, 19.3312) (-57.2912, 18.5301) (-56.3782, 17.7095) (-55.3666, 16.8695) (-54.2577, 16.0111) (-53.0526, 15.1344) (-51.7526, 14.2409) (-50.3592, 13.3299) (-48.8738, 12.4038) (-47.298, 11.4617) (-45.6338, 10.505) (-43.8825, 9.5343) (-42.0461, 8.5507) (-40.1269, 7.5533) (-38.1263, 6.5449) (-36.0471, 5.5239) (-33.8906, 4.4923) (-31.6599, 3.4499) (-29.357, 2.3971) (-26.984, 1.3354) (-24.5438, 0.2632) (-22.0383, -0.8166) (-19.471, -1.906) (-16.8437, -3.0029) (-14.1593, -4.1082) (-11.4212, -5.2214) (-8.6309, -6.3414) (-5.7928, -7.469) (-2.9088, -8.6035) (0.0179, -9.7443) (2.9842, -10.892) (5.987, -12.0462) (9.0236, -13.2057) (12.092, -14.3726) (15.1882, -15.5434) (18.3152, -16.7253) (21.4812, -17.9103) (24.6635, -19.0927) (27.8663, -20.2726) (31.0817, -21.4491) (34.3073, -22.6218) (37.5395, -23.7899) (40.7748, -24.9525) (44.0098, -26.1096) (47.2415, -27.2595) (50.4662, -28.4031) (53.6809, -29.538) (56.8819, -30.665) (60.066, -31.7825) (63.2306, -32.8894) (66.3713, -33.9861) (69.4856, -35.0708) (72.5705, -36.1425) (75.6225, -37.2017) (78.6384, -38.2458) (81.6156, -39.2754) (84.5505, -40.2888) (87.4406, -41.2851) (90.2827, -42.2636) (93.0744, -43.2238) (95.8119, -44.1643) (98.4934, -45.0842) (101.1158, -45.9827) (103.6762, -46.8595) (106.1724, -47.7125) (108.6017, -48.5424) (110.9617, -49.347) (113.2496, -50.127) (115.4637, -50.88) (117.6013, -51.6067) (119.6602, -52.3054) (121.6385, -52.9761) (123.5339, -53.6175) (125.3446, -54.2302) (127.0687, -54.8119) (128.7042, -55.3637) (130.2495, -55.8844) (131.7033, -56.373) (133.0634, -56.8302) (134.329, -57.2551) (135.4983, -57.6468) (136.57, -58.006) (137.5435, -58.3313) (138.4168, -58.6236) (139.1901, -58.8815) (139.8614, -59.1056) (140.431, -59.2957) (140.8956, -59.4501) (141.3367, -59.5977) (141.5982, -59.6843) (141.7539, -59.7362) (141.7858, -59.7469) knots 0 0 0 0 0 0.003306 0.005253 0.00752 0.010062 0.01285 0.015861 0.019079 0.022488 0.026078 0.029837 0.033757 0.037828 0.042045 0.046398 0.050884 0.055494 0.060224 0.065069 0.070023 0.075082 0.080241 0.085495 0.090841 0.096274 0.101791 0.107386 0.113057 0.118799 0.124609 0.130484 0.136419 0.142412 0.148458 0.154554 0.160697 0.166884 0.17311 0.179374 0.185671 0.191998 0.198352 0.20473 0.211128 0.217543 0.223972 0.230412 0.23686 0.243312 0.249765 0.256217 0.262663 0.2691 0.275526 0.281941 0.288345 0.294734 0.301105 0.307451 0.313767 0.320049 0.326294 0.332498 0.338659 0.344773 0.350837 0.356848 0.362801 0.368695 0.374525 0.380288 0.38598 0.391599 0.39714 0.4026 0.407976 0.413263 0.418458 0.423557 0.428556 0.433452 0.438241 0.442917 0.447478 0.451919 0.456236 0.460425 0.464482 0.468403 0.472185 0.475825 0.479322 0.482675 0.485889 0.48897 0.49193 0.494788 0.497572 0.50031 0.503032 0.505769 0.508552 0.511409 0.514365 0.517441 0.520647 0.523991 0.527474 0.531098 0.534861 0.538758 0.542789 0.546947 0.551231 0.555634 0.560154 0.564786 0.569527 0.574371 0.579315 0.584356 0.58949 0.594712 0.60002 0.605409 0.610877 0.61642 0.622034 0.627716 0.633463 0.639271 0.645138 0.651061 0.657035 0.663059 0.669128 0.675241 0.681393 0.687582 0.693804 0.700057 0.706341 0.712655 0.718998 0.725365 0.731751 0.738149 0.744556 0.750969 0.757385 0.7638 0.770211 0.776616 0.783011 0.789393 0.795759 0.802106 0.808429 0.814727 0.820996 0.827232 0.833433 0.839595 0.845714 0.851788 0.857813 0.863785 0.869702 0.875558 0.881352 0.887078 0.892735 0.898316 0.90382 0.909242 0.914577 0.919822 0.924972 0.930023 0.93497 0.939808 0.944533 0.949139 0.95362 0.95797 0.962183 0.966252 0.970169 0.973927 0.977515 0.980924 0.984141 0.987151 0.989939 0.99248 0.994747 0.996694 1 1 1 1 1
  circle A0 centre (0, 0) radius 5.15
  line L0 (-47.1, 17.9) -> (-36.9, 17.9)
  line L1 (-36.9, 17.9) -> (-36.9, 22.1)
  line L2 (-36.9, 22.1) -> (-47.1, 22.1)
  line L3 (-47.1, 22.1) -> (-47.1, 17.9)
  line L4 (-47.1, 17.9) -> (-36.9, 22.1) construction
  line L5 (-36.9, 17.9) -> (-47.1, 22.1) construction
  line L6 (-27.08, 14.1) -> (-16.88, 14.1)
  line L7 (-16.88, 14.1) -> (-16.88, 9.9)
  line L8 (-16.88, 9.9) -> (-27.08, 9.9)
  line L9 (-27.08, 9.9) -> (-27.08, 14.1)
  line L10 (-27.08, 14.1) -> (-16.88, 9.9) construction
  line L11 (-16.88, 14.1) -> (-27.08, 9.9) construction
  line L12 (65.1, -17.9) -> (54.9, -17.9)
  line L13 (54.9, -17.9) -> (54.9, -22.1)
  line L14 (54.9, -22.1) -> (65.1, -22.1)
  line L15 (65.1, -22.1) -> (65.1, -17.9)
  line L16 (65.1, -17.9) -> (54.9, -22.1) construction
  line L17 (54.9, -17.9) -> (65.1, -22.1) construction
  line L18 (29.9, -9) -> (40.1, -9)
  line L19 (40.1, -9) -> (40.1, -13.2)
  line L20 (40.1, -13.2) -> (29.9, -13.2)
  line L21 (29.9, -13.2) -> (29.9, -9)
  line L22 (29.9, -9) -> (40.1, -13.2) construction
  line L23 (40.1, -9) -> (29.9, -13.2) construction
  point P0 (0, 0)
  point P1 (141.6057, -59.6212)
  point P2 (141.3806, -59.4643)
  point P3 (141.0658, -59.2451)
  point P4 (140.6616, -58.9636)
  point P5 (140.168, -58.6208)
  point P6 (139.5855, -58.2168)
  point P7 (138.9144, -57.7525)
  point P8 (138.1554, -57.2284)
  point P9 (137.3089, -56.6459)
  point P10 (136.3756, -56.0052)
  point P11 (135.3562, -55.3078)
  point P12 (134.2513, -54.5546)
  point P13 (133.0621, -53.7467)
  point P14 (131.789, -52.8856)
  point P15 (130.4333, -51.9725)
  point P16 (128.9961, -51.0089)
  point P17 (127.4783, -49.9958)
  point P18 (125.8812, -48.9352)
  point P19 (124.2061, -47.8286)
  point P20 (122.4543, -46.6776)
  point P21 (120.6271, -45.4836)
  point P22 (118.7264, -44.2485)
  point P23 (116.7532, -42.9741)
  point P24 (114.7097, -41.6624)
  point P25 (112.5971, -40.3147)
  point P26 (110.4176, -38.9334)
  point P27 (108.1727, -37.5199)
  point P28 (105.8648, -36.0767)
  point P29 (103.4952, -34.6053)
  point P30 (101.0665, -33.1079)
  point P31 (98.5807, -31.5865)
  point P32 (96.0399, -30.0431)
  point P33 (93.4463, -28.4796)
  point P34 (90.8025, -26.8982)
  point P35 (88.1103, -25.3011)
  point P36 (85.3726, -23.6902)
  point P37 (82.5918, -22.0678)
  point P38 (79.7701, -20.4359)
  point P39 (76.9103, -18.7967)
  point P40 (74.0148, -17.1522)
  point P41 (71.0864, -15.5046)
  point P42 (68.1279, -13.8563)
  point P43 (65.1415, -12.2093)
  point P44 (62.1306, -10.5659)
  point P45 (59.0974, -8.9278)
  point P46 (56.045, -7.2978)
  point P47 (52.9761, -5.6776)
  point P48 (49.8937, -4.0696)
  point P49 (46.8004, -2.4756)
  point P50 (43.6994, -0.8981)
  point P51 (40.5932, 0.6607)
  point P52 (37.4851, 2.1994)
  point P53 (34.3778, 3.7154)
  point P54 (31.2744, 5.2068)
  point P55 (28.1777, 6.6715)
  point P56 (25.0752, 8.1131)
  point P57 (21.9724, 9.5227)
  point P58 (18.8825, 10.8937)
  point P59 (15.8082, 12.2244)
  point P60 (12.753, 13.5133)
  point P61 (9.7203, 14.7591)
  point P62 (6.713, 15.96)
  point P63 (3.7342, 17.1155)
  point P64 (0.7875, 18.2236)
  point P65 (-2.1243, 19.2839)
  point P66 (-4.9978, 20.2951)
  point P67 (-7.83, 21.2568)
  point P68 (-10.6177, 22.1677)
  point P69 (-13.358, 23.0276)
  point P70 (-16.0476, 23.8358)
  point P71 (-18.6834, 24.5921)
  point P72 (-21.2628, 25.296)
  point P73 (-23.7825, 25.9475)
  point P74 (-26.2397, 26.5464)
  point P75 (-28.6319, 27.093)
  point P76 (-30.9561, 27.587)
  point P77 (-33.2096, 28.029)
  point P78 (-35.3899, 28.419)
  point P79 (-37.4947, 28.7573)
  point P80 (-39.5211, 29.0448)
  point P81 (-41.4672, 29.2814)
  point P82 (-43.3306, 29.4679)
  point P83 (-45.1093, 29.6052)
  point P84 (-46.8012, 29.6934)
  point P85 (-48.4043, 29.7335)
  point P86 (-49.9169, 29.7263)
  point P87 (-51.3375, 29.672)
  point P88 (-52.6642, 29.5716)
  point P89 (-53.896, 29.4259)
  point P90 (-55.0312, 29.2355)
  point P91 (-56.0689, 29.0008)
  point P92 (-57.0082, 28.7231)
  point P93 (-57.8477, 28.4021)
  point P94 (-58.5873, 28.0389)
  point P95 (-59.226, 27.6343)
  point P96 (-59.7634, 27.1881)
  point P97 (-60.1991, 26.701)
  point P98 (-60.5333, 26.1735)
  point P99 (-60.7653, 25.6058)
  point P100 (-60.8934, 25.006)
  point P101 (-60.9149, 24.382)
  point P102 (-60.8305, 23.7344)
  point P103 (-60.6405, 23.0633)
  point P104 (-60.3454, 22.3691)
  point P105 (-59.9456, 21.6526)
  point P106 (-59.4419, 20.9137)
  point P107 (-58.8353, 20.1531)
  point P108 (-58.1264, 19.3714)
  point P109 (-57.3163, 18.5692)
  point P110 (-56.4059, 17.7472)
  point P111 (-55.3964, 16.9058)
  point P112 (-54.289, 16.0458)
  point P113 (-53.085, 15.1678)
  point P114 (-51.7859, 14.2727)
  point P115 (-50.393, 13.3606)
  point P116 (-48.908, 12.4329)
  point P117 (-47.3325, 11.4897)
  point P118 (-45.6682, 10.5317)
  point P119 (-43.9167, 9.5599)
  point P120 (-42.0802, 8.5749)
  point P121 (-40.1604, 7.5768)
  point P122 (-38.1595, 6.567)
  point P123 (-36.0797, 5.5453)
  point P124 (-33.9227, 4.5125)
  point P125 (-31.6912, 3.4692)
  point P126 (-29.3874, 2.4156)
  point P127 (-27.0136, 1.3526)
  point P128 (-24.5724, 0.28)
  point P129 (-22.0661, -0.8012)
  point P130 (-19.4976, -1.8911)
  point P131 (-16.8694, -2.9891)
  point P132 (-14.1839, -4.0952)
  point P133 (-11.4445, -5.209)
  point P134 (-8.6533, -6.3301)
  point P135 (-5.8138, -7.4584)
  point P136 (-2.9286, -8.5936)
  point P137 (-0.0006, -9.7353)
  point P138 (2.9671, -10.8838)
  point P139 (5.9712, -12.0385)
  point P140 (9.0089, -13.1991)
  point P141 (12.077, -14.3655)
  point P142 (15.1724, -15.5373)
  point P143 (18.3022, -16.7181)
  point P144 (21.4698, -17.9043)
  point P145 (24.657, -19.0882)
  point P146 (27.8612, -20.2691)
  point P147 (31.0784, -21.4463)
  point P148 (34.3055, -22.6197)
  point P149 (37.5393, -23.7885)
  point P150 (40.7762, -24.9519)
  point P151 (44.0129, -26.1094)
  point P152 (47.2461, -27.2603)
  point P153 (50.4726, -28.4043)
  point P154 (53.6888, -29.5401)
  point P155 (56.8914, -30.6676)
  point P156 (60.0772, -31.7857)
  point P157 (63.2433, -32.8934)
  point P158 (66.3857, -33.9905)
  point P159 (69.5016, -35.0758)
  point P160 (72.5881, -36.1483)
  point P161 (75.6417, -37.2078)
  point P162 (78.6591, -38.2527)
  point P163 (81.6378, -39.2827)
  point P164 (84.5743, -40.2967)
  point P165 (87.4659, -41.2935)
  point P166 (90.3095, -42.2726)
  point P167 (93.1025, -43.2332)
  point P168 (95.8416, -44.1742)
  point P169 (98.5244, -45.0946)
  point P170 (101.1483, -45.9937)
  point P171 (103.7101, -46.8707)
  point P172 (106.2075, -47.7244)
  point P173 (108.6381, -48.5545)
  point P174 (110.9993, -49.3598)
  point P175 (113.2886, -50.1399)
  point P176 (115.5038, -50.8935)
  point P177 (117.6425, -51.6204)
  point P178 (119.7026, -52.3196)
  point P179 (121.6819, -52.9906)
  point P180 (123.5784, -53.6325)
  point P181 (125.39, -54.2452)
  point P182 (127.115, -54.8275)
  point P183 (128.7515, -55.3795)
  point P184 (130.2977, -55.9004)
  point P185 (131.7522, -56.3895)
  point P186 (133.1132, -56.8468)
  point P187 (134.3795, -57.2719)
  point P188 (135.5495, -57.664)
  point P189 (136.622, -58.0232)
  point P190 (137.5959, -58.3489)
  point P191 (138.47, -58.6412)
  point P192 (139.2437, -58.8994)
  point P193 (139.916, -59.1238)
  point P194 (140.4859, -59.3139)
  point P195 (140.9533, -59.4696)
  point P196 (141.3172, -59.591)
  point P197 (141.5775, -59.6775)
  point P198 (141.7337, -59.7295)
  point P199 (-42, 20)
  dimension "d27" = 10.3
  dimension "d28" = 65.94
  dimension "d118" = 10.2
  dimension "d119" = 4.2
  dimension "d120" = 10.2
  dimension "d121" = 4.2
  dimension "d124" = 0
  dimension "d178" = 42
  dimension "d179" = 20
  dimension "d180" = 21.98
  dimension "d181" = 12
  dimension "d291" = 10.2
  dimension "d292" = 4.2
  dimension "d293" = 60
  dimension "d294" = 20
  dimension "d295" = 10.2
  dimension "d296" = 4.2
  dimension "d297" = 35
  dimension "d298" = 11.1
  constraints: 48 end point, 8 midpoint, 8 parallel, 4 horizontal, 4 perpendicular, 1 centre point, 201 other
  measures "d27" diameter of A0
  measures "d28" distance of A0.centre point (-60.765, 25.606)
  measures "d118" distance of L2.end L1.end
  measures "d119" distance of L1.end L0.end
  measures "d120" distance of L7.end L8.end
  measures "d121" distance of L6.end L7.end
  measures "d124" distance of A0.centre point (0, 0)
  measures "d178" horizontal distance of point (0, 0) point (-42, 20)
  measures "d179" vertical distance of point (0, 0) point (-42, 20)
  measures "d180" horizontal distance of point (0, 0) point (-21.98, 12)
  measures "d181" vertical distance of A0.centre point (-21.98, 12)
  measures "d291" distance of L14.end L13.end
  measures "d292" distance of L13.end L12.end
  measures "d293" horizontal distance of point (60, -20) point (0, 0)
  measures "d294" vertical distance of point (0, 0) point (60, -20)
  measures "d295" distance of L19.end L20.end
  measures "d296" distance of L18.end L19.end
  measures "d297" horizontal distance of point (0, 0) point (35, -11.1)
  measures "d298" vertical distance of point (0, 0) point (35, -11.1)